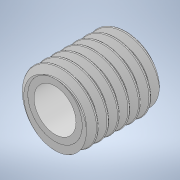
# Autodesk Inventor part: thread-m
Saved by Autodesk Inventor 2022 (Build 260153000, 153)
## iProperties
Created: 2021-10-07
Part Number: thread-m
Material: Generic
Document SubType Name: Modeling
Designer: tecware
Density: 1 g/cm^3
Appearance: Default
Author: tecware
## iProperties of the stored document thread-m_3DPrint.ipt
Created: 2021-10-07
Part Number: thread-m_3DPrint
Material: Generic
Document SubType Name: Modeling
Designer: tecware
Density: 1 g/cm^3
Appearance: Default
Author: tecware
Autodesk Inventor part; units mm, degrees
ref_plane "YZ Plane" through (0, 0, 0) normal (1, 0, 0) x (0, 1, 0)
ref_plane "XZ Plane" through (0, 0, 0) normal (0, 1, 0) x (-1, 0, 0)
ref_plane "XY Plane" through (0, 0, 0) normal (0, 0, 1) x (1, 0, 0)
sketch "Sketch1" plane through (0, 0, 0) normal (0, 0, 1) x (1, 0, 0)
  circle A0 centre (0, 0) radius 10
  circle A1 centre (0, 0) radius 6
  dimension "d0" = 20
  dimension "d46" = 12
  constraints: 2 centre point, 2 coincident
  measures "d0" diameter of A0
  measures "d46" diameter of A1
extrude "Extrusion1" add sketch "Sketch1" along normal blind 20
thread "Thread4" size "M22x3" class "6g" standard "ANSI Metric M Profile" full length
sketch "Sketch12" plane through (0, 0, 20) normal (-1, 0, 0) x (0, 1, 0)
  line L0 (10, 0) -> (10, 20)
  line L1 (10, 20) -> (7.7756, 20)
  line L2 (7.7756, 20) -> (7.7756, 0)
  line L3 (7.7756, 0) -> (10, 0)
  line L4 (0, -4) -> (0, 24) projected
  constraints: 8 end point
revolve "Revolution7" cut sketch "Sketch12" angle 360 about axis through (0, 0, 20) along (0, 0, -1)
sketch "Sketch13" plane through (0, 0, 20) normal (-1, 0, 0) x (0, 1, 0)
  line L0 (10, 0) -> (10, 20)
  line L1 (10, 20) -> (7.7756, 20)
  line L2 (7.7756, 20) -> (7.7756, 0)
  line L3 (7.7756, 0) -> (10, 0)
  line L4 (0, -4) -> (0, 24) projected
  constraints: 8 end point
revolve "Revolution8" add sketch "Sketch13" angle 360 about axis through (0, 0, 20) along (0, 0, -1) separate body
sketch "Sketch11" plane through (0, 0, 20) normal (1, 0, 0) x (0, 0, -1)
  line L0 (-1.7501, -7.9275) -> (-1.5001, -7.9275) construction
  line L1 (0.2499, -9.8485) -> (-0.0001, -10.3287) construction
  line L2 (-3.0001, -10.3287) -> (-3.2501, -9.8485) construction
  line L3 (-1.2501, -7.9275) -> (-1.5001, -7.4472) construction
  line L4 (-1.5001, -7.4472) -> (-1.7501, -7.9275) construction
  line L5 (-3.0001, -10.3287) -> (-2.7501, -9.8485) construction
  line L6 (-1.2501, -7.9275) -> (-0.2501, -9.8485)
  line L7 (-3.2501, -9.8485) -> (-2.7501, -9.8485) construction
  arc A0 (-3.2501, -9.8485) -> (-3.0001, -10.0002) centre (-3.0001, -9.7183) ccw construction
  line L8 (0.2499, -9.8485) -> (-0.2501, -9.8485) construction
  line L9 (-3.0001, -10.3287) -> (-3.0001, -9.8485) construction
  line L10 (-0.0001, -10.3287) -> (-0.0001, -9.8485) construction
  line L11 (-1.5001, -7.4472) -> (-1.5001, -7.7758) construction
  line L12 (-3.0001, -10.0002) -> (-0.0001, -10.0002)
  arc A1 (-3.0001, -10.0002) -> (-2.7501, -9.8485) centre (-3.0001, -9.7183) ccw
  line L13 (-0.2501, -9.8485) -> (-0.0001, -10.3287) construction
  line L14 (-2.7501, -9.8485) -> (-1.7501, -7.9275)
  line L15 (-0.0001, -0.0002) -> (-0.0001, 0.0177)
  line L16 (-0.0001, 0.0177) -> (-0.0001, -0.0002)
  line L17 (-0.0001, -0.0002) -> (0.0334, -0.0002)
  arc A2 (-0.2501, -9.8485) -> (-0.0001, -10.0002) centre (-0.0001, -9.7183) ccw
  arc A3 (-0.0001, -10.0002) -> (0.2499, -9.8485) centre (-0.0001, -9.7183) ccw construction
  arc A4 (-1.5001, -7.7758) -> (-1.7501, -7.9275) centre (-1.5001, -8.0576) ccw
  arc A5 (-1.2501, -7.9275) -> (-1.5001, -7.7758) centre (-1.5001, -8.0576) ccw
  line L18 (-1.5001, -7.7758) -> (-1.5001, -7.9275) construction
  line L19 (-1.5001, -7.9275) -> (-1.2501, -7.9275) construction
  dimension "d70" = 55
  dimension "d71" = 0.4803
  dimension "d72" = 0.4803
  dimension "Sketch11_ThreadOffset" = 0
  dimension "Sketch11_MajorRadius" = 10
  dimension "d75" = 3
  dimension "Sketch11_MinorRadius" = 7.7756
  constraints: 40 end point, 12 point on circle, 10 parallel, 8 tangent, 6 centre point, 6 collinear, 2 midpoint, 2 point on line, 1 horizontal, 1 perpendicular, 3 other
  measures "d70" angle of L6 L14
  measures "d71" distance of L3.end L0.end
  measures "d72" distance of L1.end L10.end
  measures "Sketch11_ThreadOffset" distance between parallel lines of L15 L10
  measures "Sketch11_MajorRadius" distance from line of L12 L15.start
  measures "d75" distance from line of L1.end L9
  measures "Sketch11_MinorRadius" distance edge to line of A5 L17
coil "Coil4" sketch "Sketch11" operation cut axis through (0, 0, 20) along (0, 0, -1) pitch 3.003 turns 8.658009 hand right bodies 2
equation "\"d70\" = d77"
equation "\"d71\" = 0.160083 * Sketch11_Pitch"
equation "\"d72\" = 0.160083 * Sketch11_Pitch"
equation "\"d75\" = Sketch11_Pitch"
equation "\"d12\" = 55deg"
equation "\"Sketch2_Pitch\" = 1.5"
equation "\"d33\" = 55deg"
equation "\"Sketch5_Pitch\" = 2.5"
equation "\"d56\" = 55deg"
equation "\"Sketch8_Pitch\" = 2.5"
equation "\"d77\" = 55deg"
equation "\"Sketch11_Pitch\" = 3"
body "Solid1"
body "Solid5"
